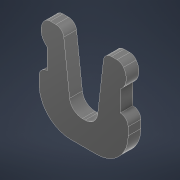
# Autodesk Inventor part: fastener_lock
Saved by Autodesk Inventor 2021 (Build 250183000, 183)
## iProperties
Created: 2021-01-30
Part Number: fastener_lock
Material: ABS Plastic
Document SubType Name: Modeling
Designer: User
Density: 1.06 g/cm^3
Appearance: Smooth - Black
Author: User
Autodesk Inventor part; units mm, degrees
ref_plane "YZ Plane" through (0, 0, 0) normal (1, 0, 0) x (0, 1, 0)
ref_plane "XZ Plane" through (0, 0, 0) normal (0, 1, 0) x (-1, 0, 0)
ref_plane "XY Plane" through (0, 0, 0) normal (0, 0, 1) x (1, 0, 0)
sketch "clip_sketch" plane through (0, 0, 0) normal (0, 0, 1) x (1, 0, 0)
  line L0 (0.2, -0.2) -> (9.8, -0.2) projected
  line L1 (9.8, -0.2) -> (9.8, 2.4) projected
  line L2 (0.2, 2.4) -> (9.8, 2.4) projected
  line L3 (0.2, -0.2) -> (0.2, 2.4) projected
  line L4 (0.4, -0.2) -> (0.4, 2.4)
  line L5 (9.6, 2.4) -> (9.6, -0.2)
  line L6 (0.4, -0.2) -> (0.4, -0.2)
  line L7 (-0.6, -1.2) -> (-0.6, -2.2)
  line L8 (3.4, -6.2) -> (6.6, -6.2)
  line L9 (10.6, -2.2) -> (10.6, -1.2)
  line L10 (9.6, -0.2) -> (9.6, -0.2)
  line L11 (0.4, 2.4) -> (0.4, 5.4)
  line L12 (0.4, 5.4) -> (9.6, 5.4)
  line L13 (9.6, 5.4) -> (9.6, 2.4)
  line L14 (3.4, -3.2) -> (2.4, 5.4)
  line L15 (6.6, -3.2) -> (7.6, 5.4)
  arc A0 (0.4, 5.4) -> (0.4, 2.4) centre (1.5, 3.9) ccw
  arc A1 (9.6, 2.4) -> (9.6, 5.4) centre (8.5, 3.9) ccw
  line L16 (5, 2.4) -> (5, -0.2) construction
  arc A2 (0.4, -0.2) -> (-0.6, -1.2) centre (0.4, -1.2) ccw
  arc A3 (10.6, -1.2) -> (9.6, -0.2) centre (9.6, -1.2) ccw
  arc A4 (-0.6, -2.2) -> (3.4, -6.2) centre (3.4, -2.2) ccw
  arc A5 (6.6, -6.2) -> (10.6, -2.2) centre (6.6, -2.2) ccw
  line L17 (3.4, -3.2) -> (6.6, -3.2)
  point P0 (0, 0)
  point P1 (-0.6, -0.2)
  dimension "d31" = 0.2
  dimension "d32" = 0.2
  dimension "d33" = 1
  dimension "d34" = 1
  dimension "d35" = 6
  dimension "d36" = 2
  dimension "d37" = 2
  dimension "d39" = 7
  dimension "d40" = 7
  dimension "d41" = 3
  dimension "d42" = 1
  dimension "d43" = 4
  dimension "d44" = 3
  dimension "d45" = 1
  constraints: 28 end point, 12 point on circle, 10 point on line, 8 perpendicular, 8 tangent, 6 centre point, 2 equal radius, 2 midpoint, 1 equal length, 1 parallel
  measures "d31" distance between parallel lines of L3 L4
  measures "d32" distance between parallel lines of L1 L5
  measures "d33" distance between parallel lines of L4 L7
  measures "d34" distance between parallel lines of L9 L5
  measures "d35" distance between parallel lines of L8 L0
  measures "d36" distance of L12.end L15.end
  measures "d37" distance of L11.end L14.end
  measures "d39" diameter of A0.centre L16
  measures "d40" diameter of A1.centre L16
  measures "d41" distance between parallel lines of L2 L12
  measures "d42" radius of A2
  measures "d43" radius of A4
  measures "d44" distance between parallel lines of L8 L17
  measures "d45" horizontal distance of L14.start L14.end
ref_plane "Work Plane1" through (0.2, -0.2, 2) normal (0, 0, -1) x (0, 1, 0)
extrude "clip" add sketch "clip_sketch" along normal blind 1.6 contours L4 L2 L14 L0 | L0 L14 L17 L15 A3 L9 A5 L8 A4 L7 A2 | L11 L12 L14 L2 | A0 L11 | L15 L2 L5 L0 | L15 L12 L13 L2 | L13 A1
fillet "teeth" radius 1 4 edges at (2.4, 5.4, 0.8) (7.6, 5.4, 0.8) (0.4, 5.4, 0.8) (9.6, 5.4, 0.8)
fillet "inside" radius 1.6 2 edges at (3.4, -3.2, 0.8) (6.6, -3.2, 0.8)
body "Solid2"
